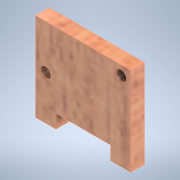
# Autodesk Inventor part: SwitchHolder_Bottom_V3
Saved by Autodesk Inventor 2022.2 (Build 262287000, 287)
## iProperties
Created: 2022-12-01
Part Number: SwitchHolder_Bottom_V3
Material: Wood (Oak)
Document SubType Name: Modeling
Designer: jaege
Density: 0.76 g/cm^3
Appearance: Red Oak - Natural Low Gloss
Author: jaege
Autodesk Inventor part; units mm, degrees
ref_plane "YZ Plane" through (0, 0, 0) normal (1, 0, 0) x (0, 1, 0)
ref_plane "XZ Plane" through (0, 0, 0) normal (0, 1, 0) x (-1, 0, 0)
ref_plane "XY Plane" through (0, 0, 0) normal (0, 0, 1) x (1, 0, 0)
sketch "Sketch1" plane through (0, 0, 0) normal (0, 0, 1) x (1, 0, 0)
  line L0 (-14, 0) -> (14, 0)
  line L1 (14, 0) -> (14, 16)
  line L2 (14, 16) -> (-14, 16)
  line L3 (-14, 16) -> (-14, 0)
  circle A0 centre (-11.1, 2.85) radius 1.55
  circle A1 centre (11.1, 13.15) radius 1.55
  line L4 (-11.1, 2.85) -> (-14, 2.85) construction
  line L5 (11.1, 13.15) -> (14, 13.15) construction
  line L6 (11.1, 13.15) -> (11.1, 16) construction
  line L7 (-11.1, 2.85) -> (-11.1, 0) construction
  line L8 (-14, 0) -> (14, 0) construction
  line L9 (14, 0) -> (14, -6)
  line L10 (14, -6) -> (8, -6) construction
  line L11 (-14, -6) -> (-14, 0)
  line L12 (-14, -6) -> (-8, -6) construction
  line L13 (-8, -6) -> (-8, -10)
  line L14 (-8, -10) -> (-14, -10)
  line L15 (-14, -10) -> (-14, -6)
  line L16 (14, -6) -> (8, -6) construction
  line L17 (8, -6) -> (8, -10)
  line L18 (8, -10) -> (14, -10)
  line L19 (14, -10) -> (14, -6)
  line L20 (-8, -6) -> (-14, -6) construction
  line L21 (8, -6) -> (-8, -6)
  point P0 (0, 0)
  point P1 (0, 0)
  point P2 (14, 0)
  point P3 (14, 0)
  dimension "d0" = 3.1
  dimension "d1" = 22.2
  dimension "d2" = 10.3
  dimension "d3" = 16
  dimension "d4" = 28
  dimension "d5" = 22
  dimension "d8" = 6
  dimension "d9" = 6
  dimension "d10" = 4
  constraints: 44 end point, 12 parallel, 8 perpendicular, 5 point on line, 4 horizontal, 2 centre point, 1 coincident, 1 collinear, 1 equal radius, 1 horizontal alignment, 1 midpoint
  measures "d0" diameter of A1
  measures "d1" horizontal distance of L5.start L4.start
  measures "d2" vertical distance of L5.start L4.start
  measures "d3" distance of L0.end L1.end
  measures "d4" distance of L1.end L2.end
  measures "d5" distance between parallel lines of L2 L10
  measures "d8" distance of L13.end L14.end
  measures "d9" distance of L18.end L17.end
  measures "d10" distance of L18.end L9.end
extrude "Extrusion1" add sketch "Sketch1" along normal blind 4
body "Solid1"
